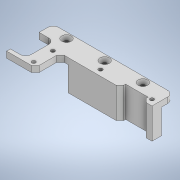
# Autodesk Inventor part: bridge_structure_A
Saved by Autodesk Inventor 2021 (Build 250183000, 183)
## iProperties
Created: 2026-02-14
Part Number: bridge_structure_A
Material: Generic
Document SubType Name: Modeling
Designer: Toby
Density: 1 g/cm^3
Appearance: Default
Author: Toby
Autodesk Inventor part; units mm, degrees
ref_plane "YZ Plane" through (0, 0, 0) normal (1, 0, 0) x (0, 1, 0)
ref_plane "XZ Plane" through (0, 0, 0) normal (0, 1, 0) x (-1, 0, 0)
ref_plane "XY Plane" through (0, 0, 0) normal (0, 0, 1) x (1, 0, 0)
sketch "Sketch1" plane through (0, 0, 0) normal (0, 0, 1) x (1, 0, 0)
  line L0 (-31.5, 8) -> (31.5, 8)
  line L1 (31.5, 8) -> (31.5, -8)
  line L2 (31.5, -8) -> (-31.5, -8)
  line L3 (-31.5, -8) -> (-31.5, 8)
  point P0 (0, 0)
  dimension "d0" = 16
  dimension "d1" = 8
  dimension "d2" = 63
  dimension "d3" = 31.5
  constraints: 8 end point, 2 parallel, 1 horizontal, 1 perpendicular
  measures "d0" distance of L2.end L0.start
  measures "d1" distance from line of point (0, 0) L0
  measures "d2" distance of L0.start L0.end
  measures "d3" distance from line of point (0, 0) L3
extrude "Extrusion1" add sketch "Sketch1" along normal blind 5
sketch "Sketch2" plane through (-31.5, 8, 0) normal (0, 1, 0) x (1, 0, 0)
  line L0 (0, 0) -> (0, -5) projected
  line L1 (63, 0) -> (0, 0) projected
  circle A0 centre (33, -2) radius 1
  circle A1 centre (60, -2) radius 1
  point P0 (31.5, 0)
  dimension "d6" = 33
  dimension "d7" = 60
  dimension "d8" = 2
  dimension "d9" = 2
  dimension "d10" = 2
  dimension "d11" = 2
  constraints: 2 centre point, 2 coincident
  measures "d6" distance from line of L0 point (33, -2)
  measures "d7" distance from line of L0 point (60, -2)
  measures "d8" distance from line of L1 point (33, -2)
  measures "d9" distance from line of L1 point (60, -2)
  measures "d10" diameter of A0
  measures "d11" diameter of A1
extrude "Extrusion2" cut sketch "Sketch2" against normal blind 16
sketch "Sketch4" plane through (0, 0, 5) normal (0, 0, 1) x (1, 0, 0)
  line L0 (-31.5, -8) -> (31.5, -8) projected
  line L1 (-31.5, -8) -> (-12.5, -8)
  line L2 (-12.5, -8) -> (-12.5, 4.8)
  line L3 (-12.5, 4.8) -> (-31.5, 4.8)
  line L4 (-31.5, 4.8) -> (-31.5, -8)
  line L5 (31.5, 8) -> (-31.5, 8) projected
  point P0 (0, 0)
  dimension "d24" = 19
  dimension "d25" = 3.2
  constraints: 8 end point, 2 parallel, 1 horizontal, 1 perpendicular
  measures "d24" distance of L2.end L3.end
  measures "d25" distance between parallel lines of L3 L5
extrude "Extrusion4" cut sketch "Sketch4" against normal blind 5
sketch "Sketch5" plane through (-31.5, 8, 0) normal (0, 1, 0) x (1, 0, 0)
  line L0 (0, 0) -> (0, -5) projected
  line L1 (0, -1.2) -> (8, -1.2)
  line L2 (8, -1.2) -> (8, -5)
  line L3 (8, -5) -> (0, -5)
  line L4 (0, -5) -> (0, -1.2)
  line L5 (63, 0) -> (0, 0) projected
  line L6 (63, -5) -> (0, -5) projected
  point P0 (31.5, 0)
  dimension "d28" = 1.2
  dimension "d29" = 8
  constraints: 8 end point, 2 parallel, 1 collinear, 1 horizontal, 1 perpendicular, 1 point on line
  measures "d28" distance between parallel lines of L1 L5
  measures "d29" distance of L2.end L3.end
extrude "Extrusion5" cut sketch "Sketch5" against normal blind 5
sketch "Sketch6" plane through (-31.5, 8, 0) normal (0, 1, 0) x (1, 0, 0)
  line L0 (8, -1.2) -> (0, -1.2) projected
  line L1 (0, -1.2) -> (10, -1.2)
  line L2 (10, -1.2) -> (10, -18.2)
  line L3 (10, -18.2) -> (0, -18.2)
  line L4 (0, -18.2) -> (0, -1.2)
  line L5 (8, -5) -> (10, -5)
  line L6 (10, -5) -> (10, -18.2)
  line L7 (10, -18.2) -> (8, -18.2)
  line L8 (8, -18.2) -> (8, -5)
  line L9 (0, -18.2) -> (8, -18.2)
  line L10 (8, -18.2) -> (8, -16.2)
  line L11 (8, -16.2) -> (0, -16.2)
  line L12 (0, -16.2) -> (0, -18.2)
  line L13 (63, -5) -> (8, -5) projected
  line L14 (8, -1.2) -> (8, -5) projected
  point P0 (31.5, 0)
  point P1 (10, -5)
  point P2 (0, -16.2)
  dimension "d32" = 2
  dimension "d33" = 15
  dimension "d34" = 2
  constraints: 24 end point, 6 parallel, 3 horizontal, 3 perpendicular, 2 collinear, 1 point on line
  measures "d32" distance between parallel lines of L2 L8
  measures "d33" distance between parallel lines of L11 L0
  measures "d34" distance between parallel lines of L3 L11
extrude "Extrusion6" add sketch "Sketch6" against normal blind 3.2 contours L5 L2 L3 L8 | L11 L8 L3 L4
sketch "Sketch7" plane through (-31.5, 8, 0) normal (0, 1, 0) x (1, 0, 0)
  line L0 (0, 0) -> (0, -1.2) projected
  line L1 (0, -16.2) -> (0, -18.2) projected
  line L2 (63, 0) -> (0, 0) projected
  circle A0 centre (12, -6) radius 1
  circle A1 centre (12, -16) radius 1
  line L3 (10, -18.2) -> (0, -18.2) projected
  line L4 (10, -5) -> (19, -5) projected
  line L5 (10, -18.2) -> (15, -18.2)
  line L6 (15, -18.2) -> (15, -5)
  line L7 (15, -5) -> (10, -5)
  line L8 (10, -5) -> (10, -18.2)
  point P0 (31.5, 0)
  point P1 (12, -5)
  dimension "d37" = 12
  dimension "d38" = 12
  dimension "d39" = 16
  dimension "d40" = 6
  dimension "d41" = 2
  dimension "d42" = 2
  dimension "d43" = 5
  constraints: 8 end point, 2 centre point, 2 coincident, 2 parallel, 1 horizontal, 1 perpendicular, 1 point on line
  measures "d37" distance from line of L0 point (12, -6)
  measures "d38" distance from line of L1 point (12, -16)
  measures "d39" distance from line of L2 point (12, -16)
  measures "d40" distance from line of L2 point (12, -6)
  measures "d41" diameter of A0
  measures "d42" diameter of A1
  measures "d43" distance between parallel lines of L8 L6
extrude "Extrusion7" add sketch "Sketch7" against normal blind 3.2
chamfer "Chamfer1" distance 2 angle 45 2 edges at (-16.5, 6.4, 18.2) (-16.5, 6.4, 5)
fillet "Fillet1" radius 3 2 edges at (-23.5, 6.4, 1.2) (-23.5, 6.4, 16.2)
sketch "Sketch10" plane through (-31.5, 8, 0) normal (0, 1, 0) x (1, 0, 0)
  line L0 (63, -5) -> (17, -5) projected
  line L1 (46.2, -5) -> (58, -5)
  line L2 (58, -5) -> (58, -2)
  line L3 (58, -2) -> (46.2, -2)
  line L4 (46.2, -2) -> (46.2, -5)
  line L5 (0, 0) -> (0, -1.2) projected
  line L6 (63, 0) -> (0, 0) projected
  point P0 (31.5, 0)
  dimension "d73" = 46.2
  dimension "d74" = 58
  dimension "d75" = 2
  constraints: 8 end point, 2 parallel, 1 horizontal, 1 perpendicular, 1 point on line
  measures "d73" distance between parallel lines of L5 L4
  measures "d74" distance from line of L5.start L2
  measures "d75" distance between parallel lines of L6 L3
extrude "Extrusion9" cut sketch "Sketch10" against normal blind 16
chamfer "Chamfer2" distance 2 angle 45 2 edges at (14.7, 0, 5) (26.5, 0, 5)
sketch "Sketch11" plane through (-31.5, 8, 0) normal (0, 1, 0) x (1, 0, 0)
  line L0 (63, 0) -> (0, 0) projected
  line L1 (0, 0) -> (63, 0)
  line L2 (63, 0) -> (63, 6.2)
  line L3 (63, 6.2) -> (0, 6.2)
  line L4 (0, 6.2) -> (0, 0)
  line L5 (63, 0) -> (63, -5) projected
  point P0 (31.5, 0)
  dimension "d81" = 6.2
  constraints: 8 end point, 2 parallel, 1 collinear, 1 horizontal, 1 perpendicular
  measures "d81" distance between parallel lines of L0 L3
extrude "Extrusion10" add sketch "Sketch11" against normal blind 3
sketch "Sketch12" plane through (-31.5, 8, 18.2) normal (0, 1, 0) x (1, 0, 0)
  line L0 (63, 24.4) -> (0, 24.4) projected
  line L1 (0, 24.4) -> (0, 17) projected
  point P0 (31.5, 18.2)
  point P1 (10, 21.4)
  point P2 (30, 21.4)
  point P3 (50, 21.4)
  dimension "d84" = 3
  dimension "d85" = 3
  dimension "d86" = 3
  dimension "d87" = 20
  dimension "d88" = 20
  dimension "d89" = 10
  measures "d84" distance from line of L0 point (10, 21.4)
  measures "d85" distance from line of L0 point (30, 21.4)
  measures "d86" distance from line of L0 point (50, 21.4)
  measures "d87" distance of point (30, 21.4) point (10, 21.4)
  measures "d88" distance of point (50, 21.4) point (30, 21.4)
  measures "d89" distance from line of L1 point (10, 21.4)
hole "Hole2" at (-21.5, 8, -3.2) at (-1.5, 8, -3.2) at (18.5, 8, -3.2) direction (0, -1, 0) diameter 2 depth 5 tip angle 118 countersink diameter 5 countersink angle 90
fillet "Fillet2" radius 3 2 edges at (31.5, 6.5, -6.2) (-31.5, 6.5, -6.2)
body "Solid1"
